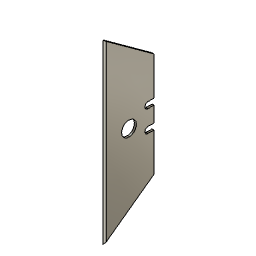
Blade (Autodesk Fusion 360 design; units mm, degrees)
Autodesk Fusion 360 part; units mm, degrees
sketch "sketch 197" plane through (0, 0, 0) normal (1, 0, 0) x (0, 0, -1)
  line L0 (-50.2206, 8.5) -> (-42.2933, -8.5) construction
  line L1 (-65.25, -8.5) -> (-52.8988, 8.5)
  line L2 (-52.8988, 8.5) -> (-17.6012, 8.5)
  line L3 (-17.6012, 8.5) -> (-5.25, -8.5)
  line L4 (-5.25, -8.5) -> (-65.25, -8.5)
  line L5 (-35.25, 8.5) -> (-35.25, -8.5) construction
  line L6 (-39.924, 8.5) -> (-39.924, 6.403)
  arc A0 (-39.924, 6.403) -> (-37.876, 6.403) centre (-38.9, 6.403) ccw
  line L7 (-37.876, 6.403) -> (-37.876, 8.5)
  line L8 (-32.624, 8.5) -> (-32.624, 6.403)
  arc A1 (-32.624, 6.403) -> (-30.576, 6.403) centre (-31.6, 6.403) ccw
  line L9 (-30.576, 6.403) -> (-30.576, 8.5)
  line L10 (-38.9, 6.403) -> (-31.6, 6.403) construction
  circle A2 centre (-35.25, 0) radius 2.5
  line L11 (46.3443, -5.345) -> (87.1281, -24.3628)
  arc A3 (80.4719, -38.6372) -> (87.1281, -24.3628) centre (83.8, -31.5) ccw
  line L12 (80.4719, -38.6372) -> (29.7186, -14.9706)
  arc A4 (29.7186, -14.9706) -> (2.2, -27.0571) centre (21.2663, -33.0967) ccw
  arc A5 (33.4, 27.1233) -> (46.3443, -5.345) centre (57.121, 17.7658) ccw
  line L13 (90.9372, -34.8281) -> (34.7461, -8.6258)
  arc A6 (-14.6883, 10.75) -> (-12.5398, 11.6563) centre (-14.6883, 13.75) ccw
  arc A7 (2.5, 18) -> (-12.5398, 11.6563) centre (2.5, -3) ccw
  line L14 (-40.996, 12.4821) -> (-43.4847, 17.8192)
  line L15 (-38.2771, 10.75) -> (-14.6883, 10.75)
  circle A8 centre (51.75, 5.6506) radius 3.7
  circle A9 centre (68.5167, -2.1678) radius 3.7
  circle A10 centre (85.2834, -9.9862) radius 3.7
  line L16 (51.75, 5.6506) -> (85.2834, -9.9862) construction
  line L17 (-35.25, 0) -> (0, 0) construction
  arc A11 (-40.996, 12.4821) -> (-38.2771, 10.75) centre (-38.2771, 13.75) ccw
extrude "Extrude1" add sketch "sketch 197" along normal mid plane 0.65 contours L1 L2 L3 L4 L6 A0 L7 L8 A1 L9
split_face "SplitFace1" 1 faces at (0.1083, -8.5, 45.25) by plane through (0, 0, 0) normal (1, 0, 0)
draft "Draft1" angle 67.5 neutral plane through (0, 0, 0) pull (1, 0, 0) 1 faces at (0.1083, -8.5, 25.25)
mirror "Mirror2" about plane through (0, 0, 0) normal (1, 0, 0) of 1 faces at (0.1083, -8.2385, 25.44)
